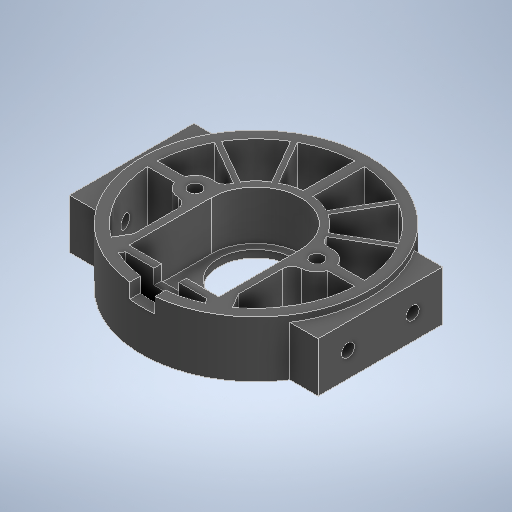
# Autodesk Inventor part: volume_case_under
Saved by Autodesk Inventor 2026.1 (Build 301233020, 233B)
## iProperties
Created: 2026-02-01
Part Number: volume_case_under
Material: 一般
Document SubType Name: Modeling
Designer: hibik
Density: 1 g/cm^3
Appearance: 既定
Author: hibik
Autodesk Inventor part; units mm, degrees
ref_plane "XZ Plane" through (0, 0, 0) normal (0, 1, 0) x (-1, 0, 0)
ref_plane "XY Plane" through (0, 0, 0) normal (0, 0, 1) x (1, 0, 0)
sketch "スケッチ1" plane through (0, 0, 0) normal (0, 1, 0) x (-1, 0, 0)
  circle A0 centre (0, 0) radius 9
  line L0 (9, 0) -> (-9, 0)
  line L1 (-9, 0) -> (-9, 16.5)
  line L2 (-9, 16.5) -> (9, 16.5)
  line L3 (9, 16.5) -> (9, 0)
  dimension "d0" = 18
  dimension "d1" = 16.5
  constraints: 8 end point, 2 parallel, 2 vertical, 1 coincident, 1 horizontal, 1 perpendicular, 3 other
  measures "d1" distance of L2.end L0.start
extrude "押し出し1" add sketch "スケッチ1" along normal blind 9.8
shell "シェル1" thickness 1.5 outward yes removed faces 1 at (-3, 9.8, 5.5)
sketch "スケッチ2" plane through (0, -1.5, 0) normal (0, -1, 0) x (1, 0, 0)
  circle A0 centre (0, 0) radius 20.8387
  circle A1 centre (0, 0) radius 23
  point P0 (10.5, 18)
  dimension "d29" = 46
  constraints: 2 coincident, 1 centre point, 3 other
  measures "d29" diameter of A1
extrude "押し出し2" add sketch "スケッチ2" against normal up to surface (11.3 mm away)
sketch "スケッチ3" plane through (0, 9.8, 0) normal (0, 1, 0) x (1, 0, 0)
  line L0 (13.3166, -18.8592) -> (9.8615, -20.8747)
  line L1 (9.8615, -20.8747) -> (7.0449, -16.0462)
  line L2 (7.0449, -16.0462) -> (10.5, -14.0307)
  line L3 (10.5, -14.0307) -> (13.3166, -18.8592)
  line L4 (10.5, -18) -> (10.5, 0) projected
  line L5 (-10.5, -18) -> (10.5, -18) projected
  circle A0 centre (0, 0) radius 23 projected
  line L6 (8.7724, -15.0385) -> (11.589, -19.8669)
  circle A1 centre (0, 0) radius 23 projected
  line L7 (0, 23) -> (1, 23)
  line L8 (1, 23) -> (1, 10.4523)
  line L9 (1, 10.4523) -> (0, 10.4523)
  line L10 (0, 10.4523) -> (0, 23)
  arc A2 (10.5, 0) -> (-10.5, 0) centre (0, 0) ccw projected
  line L11 (9, -16.5) -> (9, 0) projected
  line L12 (9, -1) -> (23, -1)
  line L13 (23, -1) -> (23, 1)
  line L14 (23, 1) -> (9, 1)
  line L15 (9, 1) -> (9, -1)
  line L16 (-0.25, 0.433) -> (0.25, -0.433)
  line L17 (0.25, -0.433) -> (20.1686, 11.067)
  line L18 (20.1686, 11.067) -> (19.6686, 11.933)
  line L19 (19.6686, 11.933) -> (-0.25, 0.433)
  line L20 (-0.433, 0.25) -> (0.433, -0.25)
  line L21 (0.433, -0.25) -> (11.933, 19.6686)
  line L22 (11.933, 19.6686) -> (11.067, 20.1686)
  line L23 (11.067, 20.1686) -> (-0.433, 0.25)
  point P0 (0, 10.5)
  point P1 (1, 22.9783)
  point P2 (11.0643, 20.1639)
  point P3 (4.811, 9.333)
  point P4 (5.6771, 8.833)
  point P5 (11.9303, 19.6639)
  point P6 (19.6639, 11.9303)
  point P7 (8.833, 5.6771)
  point P8 (9.333, 4.811)
  point P9 (20.1639, 11.0643)
  point P10 (22.9783, 1)
  point P11 (10.4523, 1)
  point P12 (10.5, -1)
  point P13 (22.9783, -1)
  point P14 (13.2727, -18.7839)
  point P15 (8.1846, -18)
  point P16 (9.8176, -20.7994)
  dimension "d8" = 4
  dimension "d9" = 1
  dimension "d10" = 2
  dimension "d11" = 30
  dimension "d12" = 60
  constraints: 42 end point, 10 parallel, 5 midpoint, 5 perpendicular, 4 point on line, 2 equal length, 2 horizontal, 2 point on circle, 1 coincident, 1 vertical, 5 other
  measures "d8" distance between parallel lines of L1 L3
  measures "d9" distance of L7.start L7.end
  measures "d10" distance of L12.end L13.end
  measures "d11" angle of L14 L17
  measures "d12" angle of L14 L21
extrude "押し出し3" add sketch "スケッチ3" against normal up to surface (11.3 mm away) contours L6 L4 L3 A0 | A0 L1 L5 L6 | L12 L4 A2 L14 A0 | A0 L8 A2 L10 | A0 L21 A2 L23 | L17 A2 L19 A0
mirror "ミラー1" about plane through (0, 9.8, -10.5) normal (-1, 0, 0) of "押し出し3"
sketch "スケッチ5" plane through (0, 0, 0) normal (0, 1, 0) x (1, 0, 0)
  circle A0 centre (0, 0) radius 10.5 construction
  line L0 (-9, -16.5) -> (9, -16.5) projected
  line L1 (-9, -10.5) -> (9, -10.5)
  line L2 (9, -10.5) -> (9, -16.5)
  line L3 (9, -16.5) -> (-9, -16.5)
  line L4 (-9, -16.5) -> (-9, -10.5)
  line L5 (-9, -16.5) -> (-9, 0) projected
  point P0 (9, 0)
  dimension "d17" = 21
  constraints: 8 end point, 2 horizontal, 2 parallel, 1 coincident, 1 horizontal alignment, 1 perpendicular, 1 point on line, 1 other
extrude "押し出し4" cut sketch "スケッチ5" against normal through all
sketch "スケッチ6" plane through (0, 0, 0) normal (0, 1, 0) x (1, 0, 0)
  circle A0 centre (0, 0) radius 7.5
  dimension "d18" = 15
  constraints: 1 centre point, 1 coincident
  measures "d18" diameter of A0
extrude "押し出し5" cut sketch "スケッチ6" against normal through all
sketch "スケッチ7" plane through (0, 9.8, 0) normal (0, 1, 0) x (-1, 0, 0)
  circle A0 centre (12.25, 0) radius 3.25
  circle A1 centre (-12.25, 0) radius 3.25
  line L0 (9, 16.5) -> (9, 0) projected
  line L1 (-9, 0) -> (-9, 16.5) projected
  point P0 (0, 0)
  dimension "d21" = 6.5
  constraints: 2 centre point, 2 horizontal alignment, 2 tangent, 1 equal radius
  measures "d21" diameter of A0
extrude "押し出し6" add sketch "スケッチ7" against normal up to surface (11.3 mm away)
sketch "スケッチ8" plane through (0, 9.8, 0) normal (0, 1, 0) x (1, 0, 0)
  arc A0 (-10.1939, 2.5169) -> (-15.3423, 1) centre (-12.25, 0) ccw projected
  arc A1 (15.3423, 1) -> (10.1939, 2.5169) centre (12.25, 0) ccw projected
  circle A2 centre (-12.25, 0) radius 1.3
  circle A3 centre (12.25, 0) radius 1.3
  point P0 (0, 0)
  dimension "d24" = 2.6
  dimension "d25" = 2.6
  constraints: 2 centre point, 2 coincident
  measures "d24" diameter of A2
  measures "d25" diameter of A3
extrude "押し出し7" cut sketch "スケッチ8" against normal through all
fillet "フィレット1" radius 2 4 edges at (10.5, 4.15, 2.7386) (-10.5, 4.15, 2.7386) (-10.1939, 4.15, -2.5169) (10.1939, 4.15, -2.5169)
sketch "スケッチ11" plane through (9, 9.8, 16.5) normal (0, 0, -1) x (-1, 0, 0)
  line L0 (11.5, 0) -> (6.5, 0)
  line L1 (6.5, 0) -> (6.5, -3)
  line L2 (6.5, -3) -> (11.5, -3)
  line L3 (11.5, -3) -> (11.5, 0)
  line L4 (0, 0) -> (18, 0) projected
  point P0 (9, -9.8)
  point P1 (9, 0)
  dimension "d40" = 5
  dimension "d41" = 3
  constraints: 8 end point, 2 midpoint, 2 parallel, 1 horizontal, 1 perpendicular
  measures "d40" distance of L1.end L2.end
  measures "d41" distance of L2.end L0.start
extrude "押し出し9" cut sketch "スケッチ11" against normal through all
sketch "スケッチ12" plane through (0, -1.5, 0) normal (0, -1, 0) x (1, 0, 0)
  line L0 (-9, 10.5) -> (-9, 16.5) projected
  line L1 (-9, 16.5) -> (9, 16.5) projected
  line L2 (9, 10.5) -> (-9, 10.5) projected
  line L3 (9, 16.5) -> (9, 10.5) projected
  point P0 (0, 0)
extrude "押し出し10" add sketch "スケッチ12" against normal up to surface (1.5 mm away)
ref_plane "作業平面3" through (25, -1.5, 0) normal (1, 0, 0) x (0, 1, 0)
ref_plane "作業平面2" through (23, -1.5, 0) normal (1, 0, 0) x (0, 1, 0)
sketch "スケッチ13" plane through (25, -1.5, 0) normal (1, 0, 0) x (0, 1, 0)
  line L0 (0, 12.5) -> (10, 12.5)
  line L1 (10, 12.5) -> (10, -12.5)
  line L2 (10, -12.5) -> (0, -12.5)
  line L3 (0, -12.5) -> (0, 12.5)
  line L4 (0, 23) -> (0, -23) projected
  point P0 (1.5, 0)
  point P1 (0, 0)
  dimension "d47" = 25
  dimension "d48" = 10
  constraints: 8 end point, 2 midpoint, 2 parallel, 1 horizontal, 1 perpendicular
  measures "d47" distance of L2.end L0.start
  measures "d48" distance of L0.start L0.end
extrude "押し出し11" add sketch "スケッチ13" against normal up to surface round surface about axis through (0, -1.5, 0) along (0, 1, 0) radius 23 far side no
sketch "スケッチ14" plane through (25, -1.5, 0) normal (1, 0, 0) x (0, 0, -1)
  circle A0 centre (-6.5, 5) radius 1.3
  circle A1 centre (6.5, 5) radius 1.3
  line L0 (-12.5, 0) -> (12.5, 0) construction
  line L1 (0, 0) -> (0, 10) construction
  line L2 (12.5, 10) -> (-12.5, 10) construction
  line L3 (12.5, 0) -> (12.5, 10) projected
  point P0 (0, 1.5)
  point P1 (0, 5)
  dimension "d52" = 2.6
  dimension "d53" = 6
  constraints: 3 midpoint, 2 centre point, 2 end point, 1 horizontal alignment, 1 other
  measures "d52" diameter of A1
  measures "d53" distance from line of L3 A1.centre
extrude "押し出し12" cut sketch "スケッチ14" against normal up to surface round surface about axis through (0, -1.5, 0) along (0, 1, 0) radius 20.8387 far side no
mirror "ミラー2" about plane through (0, 0, 0) normal (1, 0, 0) of "押し出し11", "押し出し12"
